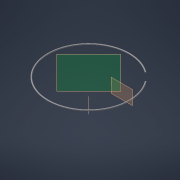
# Autodesk Inventor part: Staicring
Saved by Autodesk Inventor 2021 (Build 250183000, 183)
## iProperties
Created: 2021-01-18
Part Number: Staicring
Material: Типовые
Document SubType Name: Modeling
Designer: Dazer
Density: 1 g/cm^3
Appearance: По умолчанию
Author: Dazer
Autodesk Inventor part; units mm, degrees
ref_plane "YZ Plane" through (0, 0, 0) normal (1, 0, 0) x (0, 1, 0)
ref_plane "XZ Plane" through (0, 0, 0) normal (0, 1, 0) x (-1, 0, 0)
ref_plane "XY Plane" through (0, 0, 0) normal (0, 0, 1) x (1, 0, 0)
ref_plane "РабПлоскость1" through (0, 0, -1.5) normal (0, 0, 1) x (1, 0, 0)
sketch "Эскиз1" plane through (0, 0, -1.5) normal (0, 0, 1) x (1, 0, 0)
  circle A0 centre (22, -18.25) radius 1.25 projected
  circle A1 centre (22, -18.25) radius 1.15
  line L0 (-53, 3.9) -> (-53, -23.4) projected
  point P0 (0, 0)
  dimension "d0" = 0.1
  constraints: 1 centre point
  measures "d0" radial gap between concentric circles of A0 A1
revolve "Вращение1" add sketch "Эскиз1" angle 360 about axis through (-53, -54.25, -1.5) along (0, -1, 0) contours A1
ref_plane "РабПлоскость2" through (-53, -11.25, -1.5) normal (0, -1, 0) x (0.7071709, 0, -0.7070426)
sketch "Эскиз2" plane through (-53, -11.25, -1.5) normal (0, -1, 0) x (0.7071709, 0, -0.7070426)
  line L0 (79.7488, 0) -> (79.7488, -5)
  line L1 (79.7488, -5) -> (70.7989, -5)
  line L2 (70.7989, -5) -> (70.7989, 5)
  line L3 (70.7989, 5) -> (79.7488, 5)
  line L4 (79.7488, 5) -> (79.7488, 0)
  point P0 (36.4195, 38.534)
  dimension "d6" = 5
  dimension "d7" = 10
  constraints: 10 end point
  measures "d6" distance of L0.start L0.end
  measures "d7" distance of L1.end L2.end
extrude "Выдавливание1" cut sketch "Эскиз2" along normal blind 10
